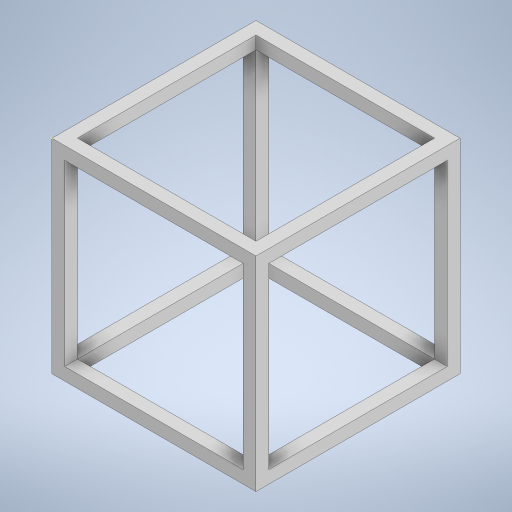
# Autodesk Inventor part: JukeBox Metal Frame
Saved by Autodesk Inventor 2024 (Build 280153000, 153)
## iProperties
Created: 2023-04-22
Part Number: JukeBox Metal Frame
Material: Generic
Document SubType Name: Modeling
Designer: newic
Density: 1 g/cm^3
Appearance: Default
Author: newic
Autodesk Inventor part; units mm, degrees
ref_plane "YZ Plane" through (0, 0, 0) normal (1, 0, 0) x (0, 1, 0)
ref_plane "XZ Plane" through (0, 0, 0) normal (0, 1, 0) x (-1, 0, 0)
ref_plane "XY Plane" through (0, 0, 0) normal (0, 0, 1) x (1, 0, 0)
sketch "Sketch3" plane through (0, 0, 0) normal (0, 0, 1) x (1, 0, 0)
  line L0 (0, 0) -> (812.8, 0) construction
  line L1 (812.8, 0) -> (812.8, -406.4) construction
  line L2 (812.8, -406.4) -> (0, -406.4) construction
  line L3 (0, -406.4) -> (0, 0) construction
  line L4 (406.4, 0) -> (0, 0)
  line L5 (0, -406.4) -> (0, 0)
  line L6 (0, -406.4) -> (406.4, -406.4)
  line L7 (406.4, 0) -> (406.4, -406.4)
  dimension "d88" = 812.8
  constraints: 8 end point, 2 midpoint, 2 perpendicular, 1 collinear, 2 other
  measures "d88" distance of L1.end L2.end
extrude "Extrusion2" add sketch "Sketch3" against normal blind 406.4
sketch "Sketch4" plane through (0, 0, 0) normal (0, 0, 1) x (1, 0, 0)
  line L0 (0, 0) -> (406.4, 0) projected
  line L1 (0, 0) -> (812.8, 0) construction
  line L2 (812.8, 0) -> (812.8, -406.4) construction
  line L3 (812.8, -406.4) -> (0, -406.4) construction
  line L4 (0, -406.4) -> (0, 0) construction
  line L5 (0, 0) -> (25.4, 0)
  line L6 (25.4, 0) -> (25.4, -25.4)
  line L7 (25.4, -25.4) -> (0, -25.4)
  line L8 (0, -25.4) -> (0, 0)
  line L9 (25.4, -25.4) -> (381, -25.4)
  line L10 (381, -25.4) -> (381, -381)
  line L11 (381, -381) -> (25.4, -381)
  line L12 (25.4, -381) -> (25.4, -25.4)
  dimension "d95" = 812.8
  dimension "d102" = 25.4
  dimension "d103" = 25.4
  dimension "d104" = 355.6
  dimension "d105" = 355.6
  constraints: 16 end point, 4 parallel, 2 horizontal, 2 perpendicular, 2 other
  measures "d95" distance of L2.end L3.end
  measures "d102" distance of L6.end L7.end
  measures "d103" distance of L5.end L6.end
  measures "d104" distance of L10.end L11.end
  measures "d105" distance of L9.end L10.end
extrude "Extrusion3" cut sketch "Sketch4" against normal blind 406.4 contours L9 L10 L11 L12
sketch "Sketch5" plane through (0, -406.4, 0) normal (-1, 0, 0) x (0, 0, 1)
  line L0 (0, 406.4) -> (-406.4, 406.4) projected
  line L1 (-406.4, 406.4) -> (-381, 406.4)
  line L2 (-381, 406.4) -> (-381, 381)
  line L3 (-381, 381) -> (-406.4, 381)
  line L4 (-406.4, 381) -> (-406.4, 406.4)
  line L5 (-381, 381) -> (-25.4, 381)
  line L6 (-25.4, 381) -> (-25.4, 25.4)
  line L7 (-25.4, 25.4) -> (-381, 25.4)
  line L8 (-381, 25.4) -> (-381, 381)
  dimension "d108" = 25.4
  dimension "d109" = 25.4
  dimension "d110" = 355.6
  dimension "d111" = 355.6
  constraints: 16 end point, 4 parallel, 2 horizontal, 2 perpendicular
  measures "d108" distance of L2.end L3.end
  measures "d109" distance of L1.end L2.end
  measures "d110" distance of L6.end L7.end
  measures "d111" distance of L5.end L6.end
extrude "Extrusion4" cut sketch "Sketch5" against normal blind 406.4 contours L5 L6 L7 L8
sketch "Sketch6" plane through (0, 0, 0) normal (0, 1, 0) x (1, 0, 0)
  line L0 (0, 406.4) -> (406.4, 406.4) projected
  line L1 (0, 406.4) -> (25.4, 406.4)
  line L2 (25.4, 406.4) -> (25.4, 381)
  line L3 (25.4, 381) -> (0, 381)
  line L4 (0, 381) -> (0, 406.4)
  line L5 (25.4, 381) -> (381, 381)
  line L6 (381, 381) -> (381, 25.4)
  line L7 (381, 25.4) -> (25.4, 25.4)
  line L8 (25.4, 25.4) -> (25.4, 381)
  point P0 (0, 0)
  dimension "d114" = 25.4
  dimension "d115" = 25.4
  dimension "d116" = 355.6
  dimension "d117" = 355.6
  constraints: 16 end point, 4 parallel, 2 horizontal, 2 perpendicular
  measures "d114" distance of L2.end L3.end
  measures "d115" distance of L1.end L2.end
  measures "d116" distance of L6.end L7.end
  measures "d117" distance of L5.end L6.end
extrude "Extrusion5" cut sketch "Sketch6" against normal blind 406.4 contours L5 L6 L7 L8
sketch "Sketch7" plane through (0, 0, 0) normal (0, 0, 1) x (1, 0, 0)
  point P0 (0, 0)
body "Solid2"
